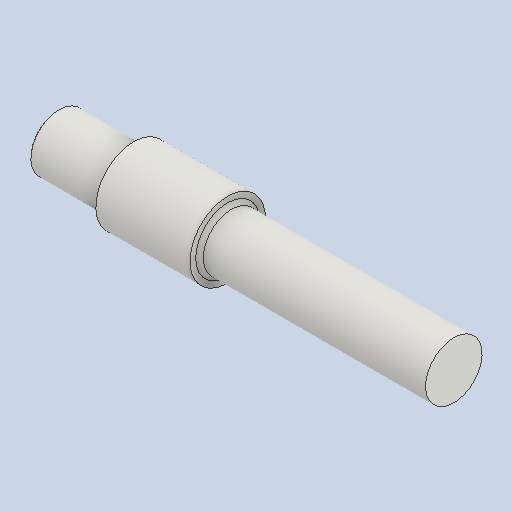
# Autodesk Inventor part: Shaft
Saved by Autodesk Inventor 2023 (Build 270158000, 158)
## iProperties
CustomPartVersion: 1
Created: 2023-01-29
Part Number: Shaft
Material: Steel
Document SubType Name: Modeling
Designer: Merve Babacan
Density: 1 g/cm^3
Appearance: Steel
Length: 210.000 mm
Author: Merve Babacan
Autodesk Inventor part; units mm, degrees
ref_plane "Start Plane" through (0, 0, 0) normal (1, 0, 0) x (0, 1, 0)
ref_plane "XZ Plane" through (0, 0, 0) normal (0, 1, 0) x (-1, 0, 0)
ref_plane "XY Plane" through (0, 0, 0) normal (0, 0, 1) x (1, 0, 0)
sketch "Main Sketch" plane through (0, 0, 0) normal (0, 0, 1) x (1, 0, 0)
  line L0 (0, 0) -> (210, 0)
  line L1 (0, 0) -> (0, 15)
  line L2 (0, 15) -> (40, 15)
  line L3 (40, 15) -> (40, 20)
  line L4 (90, 20) -> (90, 15)
  line L5 (40, 20) -> (90, 20)
  line L6 (210, 15) -> (210, 0)
  line L7 (90, 15) -> (210, 15)
  dimension "d3" = 30
  dimension "d4" = 40
  dimension "d5" = 30
  constraints: 16 end point, 5 horizontal, 4 vertical
  measures "d3" diameter of L2 L0
  measures "d4" diameter of L5 L0
  measures "d5" diameter of L7 L0
revolve "Revolution1" add sketch "Main Sketch" angle 360 about axis through (0, 0, 0) along (1, 0, 0)
chamfer "Chamfer3" distance 2 angle 45 1 edges at (40, -15, 0) measured on face at (26.6667, 14.8058, -2.4062)
chamfer "Chamfer1" distance 0.5 angle 45 1 edges at (0, -15, 0) measured on face at (25.3333, 14.9514, -1.207)
chamfer "Chamfer2" distance 2 angle 45 1 edges at (90, -15, 0) measured on face at (170, 14.9514, -1.207)
equation "\"Length\" = 210"
body "Solid1"
